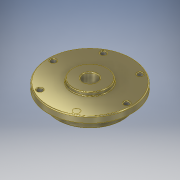
# Autodesk Inventor part: Crankcase Cover
Saved by Autodesk Inventor 2017 (Build 210142000, 142)
## iProperties
Created: 2020-01-13
Part Number: Crankcase Cover
Material: Gold
Document SubType Name: Modeling
Designer: Admin
Density: 19.3 g/cm^3
Appearance: Gold - Metal
Mass: 130.686 g
Surface Area: 32.9652 cm^2
Volume: 6.77128 cm^3
Author: Admin
Autodesk Inventor part; units mm, degrees
ref_plane "YZ Plane" through (0, 0, 0) normal (1, 0, 0) x (0, 1, 0)
ref_plane "XZ Plane" through (0, 0, 0) normal (0, 1, 0) x (-1, 0, 0)
ref_plane "XY Plane" through (0, 0, 0) normal (0, 0, 1) x (1, 0, 0)
sketch "Sketch1" plane through (0, 0, 0) normal (0, 1, 0) x (-1, 0, 0)
  circle A0 centre (0, 0) radius 19.05
  dimension "d0" = 38.1
  constraints: 1 centre point, 1 coincident
  measures "d0" diameter of A0
extrude "Extrusion1" add sketch "Sketch1" along normal mid plane 9.525
sketch "Sketch2" plane through (0, 4.7625, 0) normal (0, 1, 0) x (1, 0, 0)
  circle A0 centre (0, 0) radius 7.9375
  circle A1 centre (0, 0) radius 19.05
  dimension "d3" = 15.875
  dimension "d4" = 38.1
  constraints: 2 centre point, 2 coincident
  measures "d3" diameter of A0
  measures "d4" diameter of A1
extrude "Extrusion2" cut sketch "Sketch2" against normal blind 1.5875
sketch "Sketch3" plane through (0, -4.7625, 0) normal (0, -1, 0) x (1, 0, 0)
  circle A0 centre (0, 0) radius 14.6844
  circle A1 centre (0, 0) radius 19.05
  dimension "d7" = 29.3687
  dimension "d8" = 38.1
  constraints: 2 centre point, 2 coincident
  measures "d7" diameter of A0
  measures "d8" diameter of A1
extrude "Extrusion3" cut sketch "Sketch3" against normal blind 4.7625
sketch "Sketch4" plane through (0, 4.7625, 0) normal (0, 1, 0) x (1, 0, 0)
  circle A0 centre (0, 0) radius 3.175
  dimension "d11" = 6.35
  constraints: 1 centre point, 1 coincident
  measures "d11" diameter of A0
extrude "Extrusion4" cut sketch "Sketch4" against normal blind 25.4
sketch "Sketch5" plane through (0, 3.175, 0) normal (0, 1, 0) x (1, 0, 0)
  point P0 (0, 0)
  point P1 (-16.6688, 0)
  point P2 (-8.3344, -14.4356)
  point P3 (8.3344, -14.4356)
  point P4 (16.6688, 0)
  point P5 (8.3344, 14.4356)
  point P6 (-8.3344, 14.4356)
  dimension "d14" = 0
  dimension "d15" = 16.6687
  dimension "d18" = 360
  constraints: 7 other
  measures "d14" vertical distance of point (0, 0) point (-16.669, 0)
  measures "d15" distance of point (0, 0) point (-16.669, 0)
hole "Hole1" at (-16.6688, 3.175, 0) at (-8.3344, 3.175, 14.4356) at (8.3344, 3.175, 14.4356) at (16.6688, 3.175, 0) at (8.3344, 3.175, -14.4356) at (-8.3344, 3.175, -14.4356) direction (0, -1, 0) diameter 2.2606 depth 25.4 tip angle 118
fillet "Fillet1" radius 0.3969 2 edges at (19.05, 3.175, 0) (19.05, 0, 0)
thread "Thread1" size "3-48 UNC" class "2B" standard "ANSI Unified Screw Threads" full length
thread "Thread2" size "3-48 UNC" class "2B" standard "ANSI Unified Screw Threads" full length
thread "Thread3" size "3-48 UNC" class "2B" standard "ANSI Unified Screw Threads" full length
thread "Thread4" size "3-48 UNC" class "2B" standard "ANSI Unified Screw Threads" full length
thread "Thread5" size "3-48 UNC" class "2B" standard "ANSI Unified Screw Threads" full length
thread "Thread6" size "3-48 UNC" class "2B" standard "ANSI Unified Screw Threads" full length
fillet "Fillet2" radius 0.3175 18 edges at (16.6688, 3.175, -1.1303) (-7.9375, 3.175, 0) (-7.9375, 4.7625, 0) (-3.175, 4.7625, 0) (8.3344, 3.175, -15.5659) (-8.3344, 3.175, -15.5659) (-16.6688, 3.175, -1.1303) (-8.3344, 3.175, 13.3053) (8.3344, 3.175, 13.3053) (-14.6844, -4.7625, 0) (8.3344, 0, 13.3053) (16.6688, 0, -1.1303) (8.3344, 0, -15.5659) (-8.3344, 0, -15.5659) (-3.175, -4.7625, 0) (-8.3344, 0, 13.3053) (-16.6688, 0, -1.1303) (-14.6844, 0, 0)
body "Solid1"
